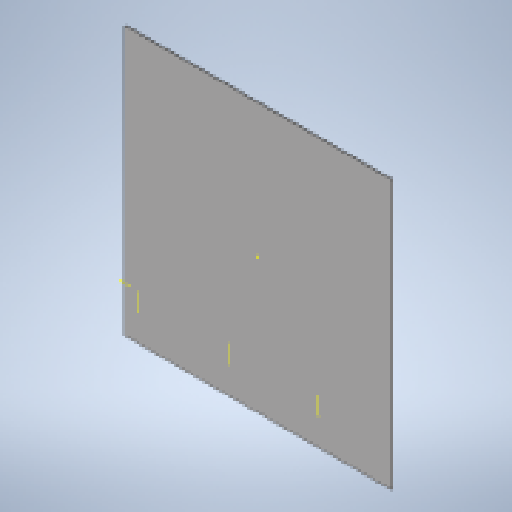
# Autodesk Inventor part: GBK 3111 shield 1
Saved by Autodesk Inventor 2026 (Build 300175000, 175)
## iProperties
Created: 2026-04-17
Part Number: GBK 3111 shield 1
Material: Steel
Document SubType Name: Sheet Metal
Designer: pokla
Stock Number: 3111
Mass: 69243.3 g
Surface Area: 44341.6 cm^2
Volume: 8820.8 cm^3
Density: 7.85 g/cm^3
Flat Pattern Width: 149 cm
Flat Pattern Length: 148 cm
Flat Pattern Area: 22052 cm^2
Sheet Metal Rule: По умолчанию_мм
Sheet Metal Width: 1490,000 мм
Sheet Metal Length: 1480,000 мм
Sheet Metal Area: 2205200,000 мм^2
Appearance: Default
Author: admin
Autodesk Inventor part; units mm, degrees
ref_plane "YZ Plane" through (0, 0, 0) normal (1, 0, 0) x (0, 1, 0)
ref_plane "XZ Plane" through (0, 0, 0) normal (0, 1, 0) x (-1, 0, 0)
ref_plane "XY Plane" through (0, 0, 0) normal (0, 0, 1) x (1, 0, 0)
sketch "Sketch1" plane through (0, 0, 0) normal (0, 0, 1) x (1, 0, 0)
  line L0 (740, -745) -> (-740, -745)
  line L1 (-740, -745) -> (-740, 745)
  line L2 (-740, 745) -> (740, 745)
  line L3 (740, 745) -> (740, -745)
  line L4 (740, -745) -> (-740, 745) construction
  line L5 (-740, -745) -> (740, 745) construction
  point P0 (0, 0)
  dimension "d0" = 1480
  dimension "d1" = 1490
  measures "d0" distance of L1.end L2.end
  measures "d1" distance of L0.end L1.end
extrude "Plate1" add sketch "Sketch1" along normal blind 4
sketch "Эскиз4" plane through (0, 0, 0) normal (0, 0, -1) x (-1, 0, 0)
  line L0 (549.4783, -556.3714) -> (549.4783, -1054.5075) construction
  line L1 (549.4783, -1054.5075) -> (509.8511, -1054.5075) construction
  line L2 (509.8511, -1054.5075) -> (509.8511, -556.3714) construction
  line L3 (509.8511, -556.3714) -> (549.4783, -556.3714) construction
  line L4 (669.2463, -498.5) -> (669.2463, -595.5) projected
  line L5 (669.2463, -595.5) -> (665.2463, -595.5) projected
  line L6 (709.6246, -495) -> (769.6246, -495) projected
  line L7 (709.6246, -495) -> (709.6246, -491) projected
  line L8 (169.3732, -498.5) -> (169.3732, -595.5) projected
  line L9 (169.3732, -595.5) -> (165.3732, -595.5) projected
  line L10 (-330.5, -498.5) -> (-330.5, -595.5) projected
  line L11 (-330.5, -595.5) -> (-334.5, -595.5) projected
  line L12 (709.6246, 1.6667) -> (769.6246, 1.6667) projected
  line L13 (709.6246, 1.6667) -> (709.6246, 5.6667) projected
  line L14 (709.6246, 498.3333) -> (769.6246, 498.3333) projected
  line L15 (709.6246, 498.3333) -> (709.6246, 502.3333) projected
  line L16 (-740, -495) -> (-710, -495) projected
  line L17 (-710, -495) -> (-710, -491) projected
  line L18 (-740, 1.6667) -> (-710, 1.6667) projected
  line L19 (-710, 1.6667) -> (-710, 5.6667) projected
  line L20 (-740, 498.3333) -> (-710, 498.3333) projected
  line L21 (-710, 498.3333) -> (-710, 502.3333) projected
  line L22 (-330.5, 709.5) -> (-330.5, 769.5) projected
  line L23 (-330.5, 709.5) -> (-334.5, 709.5) projected
  line L24 (169.3732, 709.5) -> (169.3732, 769.5) projected
  line L25 (169.3732, 709.5) -> (165.3732, 709.5) projected
  line L26 (669.2463, 709.5) -> (669.2463, 769.5) projected
  line L27 (669.2463, 709.5) -> (665.2463, 709.5) projected
  point P0 (0, 0)
  constraints: 2 other
mark "Маркировка3"
equation "\"d0\" = Лист_ширина"
equation "\"d1\" = 0.5 * Лист_длина"
equation "\"d2\" = Thickness"
equation "\"BendRadius\" = Thickness"
equation "\"BendReliefWidth\" = Thickness"
equation "\"BendReliefDepth\" = 0.5 * Thickness"
equation "\"CornerReliefSize\" = 4 * Thickness"
equation "\"MinimumRemnant\" = 2 * Thickness"
equation "\"TransitionRadius\" = BendRadius"
equation "\"JacobiRadiusSize\" = BendRadius"
equation "\"GapSize\" = Thickness"
equation "\"Лист_ширина\" = 1480"
equation "\"Лист_длина\" = 2980"
equation "\"Thickness\" = 4"
body "Solid1"
